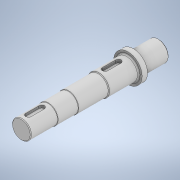
# Autodesk Inventor part: Truc_2
Saved by Autodesk Inventor 2022 (Build 260153000, 153)
## iProperties
Created: 2022-12-09
Part Number: Truc_2
Material: Generic
Document SubType Name: Modeling
Designer: nguye
Density: 1 g/cm^3
Appearance: Default
Author: nguye
Autodesk Inventor part; units mm, degrees
ref_plane "YZ Plane" through (0, 0, 0) normal (1, 0, 0) x (0, 1, 0)
ref_plane "XY Plane" through (0, 0, 0) normal (0, 0, 1) x (1, 0, 0)
sketch "Sketch1" plane through (0, 0, 0) normal (1, 0, 0) x (0, 1, 0)
  line L0 (0, 0) -> (14, 0)
  line L1 (14, 0) -> (14, -40)
  line L2 (14, -40) -> (14.5, -40)
  line L3 (14.5, -40) -> (14.5, -70)
  line L4 (14.5, -70) -> (15, -70)
  line L5 (15, -70) -> (15, -114.5)
  line L6 (15, -114.5) -> (16, -114.5)
  line L7 (16, -114.5) -> (16, -157.7226)
  line L8 (16, -157.7226) -> (21, -157.7226)
  line L9 (21, -157.7226) -> (21, -165.7226)
  line L10 (21, -165.7226) -> (15, -165.7226)
  line L11 (15, -165.7226) -> (15, -203.2226)
  line L12 (0, -243.8671) -> (0, 40.6445) projected
  line L13 (15, -203.2226) -> (0, -203.2226)
  dimension "d0" = 40
  dimension "d1" = 14
  dimension "d2" = 30
  dimension "d3" = 14.5
  dimension "d4" = 15
  dimension "d5" = 44.5
  dimension "d9" = 16
  dimension "d10" = 21
  dimension "d11" = 8
  dimension "d12" = 37.5
  dimension "d14" = 43.2226
  dimension "d24" = 15
  constraints: 26 end point, 10 perpendicular, 2 horizontal, 1 point on line, 1 vertical
  measures "d0" distance of L0.end L1.end
  measures "d1" distance of L0.start L0.end
  measures "d2" distance of L2.end L3.end
  measures "d3" distance from line of L0.start L3
  measures "d4" distance from line of L0.start L5
  measures "d5" distance of L4.end L5.end
  measures "d9" distance from line of L0.start L7
  measures "d10" distance from line of L0.start L9
  measures "d11" distance of L8.end L9.end
  measures "d12" distance of L10.end L11.end
  measures "d14" distance between parallel lines of L6 L8
  measures "d24" distance from line of L0.start L11
revolve "Revolution1" add sketch "Sketch1" angle 360 about axis through (0, 0, -10) along (0, 0, 1)
chamfer "Chamfer1" distance 1 angle 45 2 edges at (0, -15, -203.2226) (0, -14, 0)
fillet "Fillet1" radius 3 1 edges at (0, -15, -165.7226)
fillet "Fillet2" radius 2 1 edges at (0, -16, -157.7226)
fillet "Fillet3" radius 1 1 edges at (0, -15, -114.5)
fillet "Fillet4" radius 0.5 2 edges at (0, -14.5, -70) (0, -14, -40)
ref_plane "Work Plane1" through (0, 14, 0) normal (0, 1, 0) x (-1, 0, 0)
sketch "Sketch2" plane through (0, 14, 0) normal (0, 1, 0) x (-1, 0, 0)
  line L0 (0, -243.8671) -> (0, 40.6445) projected
  line L1 (0, -10) -> (0, -30) construction
  line L2 (-4, -10) -> (-4, -30)
  line L3 (4, -30) -> (4, -10)
  arc A0 (4, -10) -> (-4, -10) centre (0, -10) ccw
  arc A1 (-4, -30) -> (4, -30) centre (0, -30) ccw
  point P0 (0, 0)
  point P1 (0, -20)
  dimension "d26" = 10
  dimension "d27" = 8
  dimension "d28" = 20
  constraints: 8 end point, 4 point on circle, 4 tangent, 2 centre point, 2 point on line, 1 midpoint, 1 parallel
  measures "d26" distance of point (0, 0) L1.start
  measures "d27" distance between parallel lines of L2 L3
  measures "d28" distance of L1.start L1.end
extrude "Extrusion1" cut sketch "Sketch2" against normal blind 4
ref_plane "Work Plane2" through (0, 16, 0) normal (0, 1, 0) x (-1, 0, 0)
sketch "Sketch3" plane through (0, 16, 0) normal (0, 1, 0) x (-1, 0, 0)
  line L0 (0, -243.8671) -> (0, 40.6445) projected
  line L1 (0, -143.5) -> (0, -123.5) construction
  line L2 (4, -143.5) -> (4, -123.5)
  line L3 (-4, -123.5) -> (-4, -143.5)
  arc A0 (-4, -143.5) -> (4, -143.5) centre (0, -143.5) ccw
  arc A1 (4, -123.5) -> (-4, -123.5) centre (0, -123.5) ccw
  line L4 (-15, -113.5) -> (15, -113.5) projected
  line L5 (-16, -114.5) -> (16, -114.5) projected
  point P0 (0, 0)
  point P1 (0, -133.5)
  dimension "d32" = 8
  dimension "d34" = 9
  dimension "d35" = 20
  constraints: 8 end point, 4 point on circle, 4 tangent, 2 centre point, 2 point on line, 1 midpoint, 1 parallel
  measures "d32" distance between parallel lines of L2 L3
  measures "d34" distance from line of L5 L1.end
  measures "d35" distance of L1.end L1.start
extrude "Extrusion2" cut sketch "Sketch3" against normal blind 5
body "Solid1"
